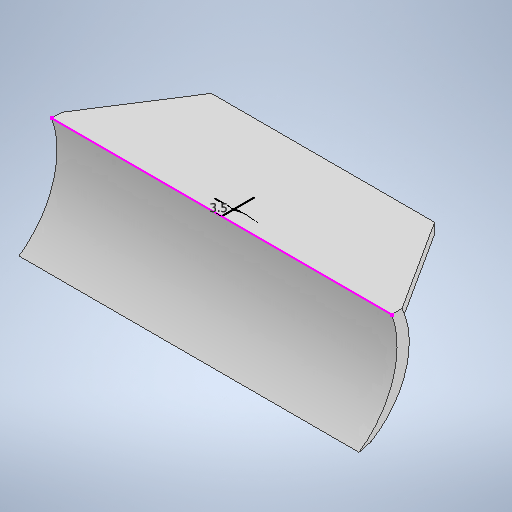
# Autodesk Inventor part: slope
Saved by Autodesk Inventor 2025.1 (Build 291241020, 241B)
## iProperties
Created: 2025-04-15
Part Number: slope
Material: Generic
Document SubType Name: Modeling
Designer: omiye
Density: 1 g/cm^3
Appearance: Default
Author: omiye
Autodesk Inventor part; units mm, degrees
ref_plane "YZ Plane" through (0, 0, 0) normal (1, 0, 0) x (0, 1, 0)
ref_plane "XZ Plane" through (0, 0, 0) normal (0, 1, 0) x (-1, 0, 0)
ref_plane "XY Plane" through (0, 0, 0) normal (0, 0, 1) x (1, 0, 0)
sketch "Sketch1" plane through (0, 0, 0) normal (0, 1, 0) x (-1, 0, 0)
  line L0 (0, 0) -> (32.5, 0)
  line L1 (32.5, 0) -> (-32.5, 0)
  line L2 (-32.5, 0) -> (-32.5, 19)
  line L3 (-32.5, 19) -> (32.5, 19)
  line L4 (32.5, 19) -> (32.5, 0)
  dimension "d0" = 32.5
  dimension "d1" = 65
  dimension "d2" = 19
  constraints: 10 end point, 2 perpendicular, 1 horizontal, 1 point on line, 1 vertical
  measures "d0" distance of L0.start L0.end
  measures "d1" distance of L0.end L1.end
  measures "d2" distance of L1.end L2.end
extrude "Extrusion1" add sketch "Sketch1" along normal blind 25
sketch "Sketch2" plane through (32.5, 0, 19) normal (1, 0, 0) x (0, 0, -1)
  line L0 (19, 0) -> (8, 0)
  line L1 (0, 0) -> (19, 0)
  line L2 (8, 0) -> (0, -2.143594)
  line L3 (0, -2.143594) -> (0, 0)
  dimension "d5" = 11
  dimension "d6" = 165
  constraints: 6 end point, 1 perpendicular, 1 point on line
  measures "d5" distance of L0.start L0.end
  measures "d6" angle of L2 L0
extrude "Extrusion2" add sketch "Sketch2" against normal up to surface (65 mm away)
sketch "Sketch3" plane through (32.5, 0, 0) normal (1, 0, 0) x (0, 0, -1)
  line L0 (-19, -2.143594) -> (-19, 25)
  line L1 (-19, 25) -> (0, 25)
  line L2 (-19, 25) -> (-19, -5)
  arc A0 (-19, -5) -> (-9.5, 25) centre (-33.73129, 16.169075) ccw
  line L3 (-19, -2.143594) -> (-11, 0)
  line L4 (-19, -5) -> (-11, 0)
  line L5 (-19, -2.143594) -> (-19, 25)
  line L6 (-19, 25) -> (-9.5, 25)
  point P0 (0, 0)
  point P1 (-14.409764, -0.913643)
  dimension "d59" = 30
  constraints: 8 end point, 2 midpoint, 2 point on circle, 1 centre point, 1 collinear, 1 perpendicular, 1 point on line
  measures "d59" distance of L0.end L2.end
extrude "Extrusion3" cut sketch "Sketch3" against normal blind 81.4375 contours L0 L1 A0 L3
sketch "Sketch4" plane through (0, 0, 0) normal (0, -1, 0) x (1, 0, 0)
  line L0 (-32.5, 0) -> (-32.5, 11) projected
  line L1 (-32.5, 0) -> (-32.5, 10.5)
  line L2 (-32.5, 10.5) -> (32.5, 10.5)
  line L3 (32.5, 11) -> (32.5, 0) projected
  line L4 (-32.5, 0) -> (-32.5, 5.25)
  line L5 (-32.5, 5.25) -> (32.5, 5.25)
  line L6 (-32.5, 5.25) -> (-18.75, 5.25)
  line L7 (-18.75, 5.25) -> (0, 5.25)
  line L8 (0, 5.25) -> (18.75, 5.25)
  line L9 (18.75, 5.25) -> (32.5, 5.25)
  circle A0 centre (18.75, 5.25) radius 1.525
  circle A1 centre (0, 5.25) radius 1.525
  circle A2 centre (-18.75, 5.25) radius 1.525
  point P0 (0, 0)
  point P1 (-17.225, 5.25)
  point P2 (-20.275, 5.25)
  point P3 (1.525, 5.25)
  point P4 (-1.525, 5.25)
  point P5 (20.275, 5.25)
  point P6 (17.225, 5.25)
  dimension "d12" = 10.5
  dimension "d13" = 5.25
  dimension "d14" = 13.75
  dimension "d15" = 18.75
  dimension "d16" = 18.75
  dimension "d17" = 3.05
  dimension "d18" = 3.05
  dimension "d19" = 3.05
  constraints: 16 end point, 5 point on line, 3 centre point, 3 coincident, 3 perpendicular, 2 midpoint
  measures "d12" distance of L0.start L1.end
  measures "d13" distance of L0.start L4.end
  measures "d14" distance of L4.end L6.end
  measures "d15" distance of L6.end L7.end
  measures "d16" distance of L7.end L8.end
  measures "d17" diameter of A0
  measures "d18" diameter of A1
  measures "d19" diameter of A2
extrude "Extrusion4" cut sketch "Sketch4" against normal blind 4 contours A2 L5 | L5 A2 | A1 L5 | L5 A1 | A0 L5 | L5 A0
sketch "Sketch5" plane through (32.5, 0, 0) normal (0, 0, -1) x (-1, 0, 0)
  line L0 (0, 25) -> (65, 25)
  line L1 (65, 25) -> (65, -2.143594)
  line L2 (0, 25) -> (65, 25)
  line L3 (65, 25) -> (65, 22)
  line L4 (65, 22) -> (0, 22)
  line L5 (0, 22) -> (0, 25)
  point P0 (32.5, 0)
  dimension "d22" = 3
  constraints: 8 end point, 2 parallel, 1 horizontal, 1 perpendicular, 1 point on line
  measures "d22" distance of L2.end L3.end
sketch "Sketch6" plane through (32.5, 0, 0) normal (1, 0, 0) x (0, 0, -1)
  line L0 (0, 0) -> (-11, 0)
  line L1 (0, 0) -> (-10, 0)
  line L2 (-11, 0) -> (0, 0)
  line L3 (-19, 25) -> (0, 25)
  arc A0 (-11, 0) -> (-6.906688, 25) centre (-24.791662, 15.093247) ccw
  line L4 (0, 0) -> (0, 25)
  line L5 (0, 25) -> (0, 22)
  line L6 (0, 22) -> (-5.548149, 22)
  line L7 (0, 0) -> (0, 2.5)
  line L8 (0, 2.5) -> (-8.68495, 2.5)
  point P0 (-9.5, 25)
  dimension "d23" = 10
  dimension "d24" = 3
  dimension "d25" = 2.5
  constraints: 10 end point, 4 point on circle, 4 point on line, 1 centre point, 1 horizontal, 1 perpendicular
  measures "d23" distance of L0.start L1.end
  measures "d24" distance of L3.end L5.end
  measures "d25" distance of L0.start L7.end
extrude "Extrusion5" cut sketch "Sketch6" against normal blind 113.5375 contours L8 A0 L6 L4
extrude "Extrusion6" add sketch "Sketch5" along normal blind 20
sketch "Sketch12" plane through (0, 25, 0) normal (0, 1, 0) x (1, 0, 0)
  line L0 (0, 0) -> (0, -9.5)
  line L1 (49.5, -9.5) -> (-49.5, -9.5)
  line L2 (0, -9.5) -> (0, 0)
  line L3 (0, -9.5) -> (0, -6)
  line L4 (0, -6) -> (8.228384, -6)
  line L5 (8.228384, -6) -> (-5.400421, -6)
  dimension "d85" = 3.5
  constraints: 10 end point, 2 point on line, 1 collinear, 1 midpoint, 1 perpendicular
  measures "d85" distance of L0.end L3.end
sketch "Sketch14" plane through (32.5, 0, 11) normal (1, 0, 0) x (0, 0, -1)
  line L0 (11, 0) -> (0, 0)
  line L1 (0, 0) -> (9.434, 0) construction
  arc A0 (-3.409764, -0.913643) -> (1.5, 25) centre (-22.73129, 16.169075) ccw
  line L2 (1.5, 25) -> (31, 25)
  arc A1 (-8.000486, -4.999258) -> (1.5, 25) centre (-22.726506, 16.168322) ccw
  line L3 (-3.409764, -0.913643) -> (0, 0)
  line L4 (-3.409764, -0.913643) -> (0, 0)
  line L5 (-8.000486, -4.999258) -> (-4.590768, -4.085627)
  line L6 (-8.000486, -4.999258) -> (-4.470486, -4.999258) construction
  line L7 (-4.590768, -4.085627) -> (0, 0)
  point P0 (28, 25)
  point P1 (-2.386043, 0.31942)
  dimension "d60" = 9.434
  dimension "d62" = 3.53
  dimension "d63" = 15
  constraints: 10 end point, 2 horizontal, 2 point on circle, 1 centre point, 1 collinear, 1 equal length
  measures "d60" distance of L0.end L5.start
  measures "d62" distance of L5.start L5.end
  measures "d63" angle of L6 L5
extrude "Extrusion12" add sketch "Sketch14" against normal up to surface (65 mm away)
sketch "Sketch15" plane through (32.5, 0, 0) normal (1, 0, 0) x (0, 0, -1)
  arc A0 (-19.000486, -4.999258) -> (-13.386043, 0.31942) centre (-33.726506, 16.168322) ccw
  line L0 (-9.5, 25) -> (20, 25)
  arc A1 (-19.000486, -4.999258) -> (-9.5, 25) centre (-33.729569, 16.169292) ccw
  line L1 (-9.5, 25) -> (-6.5, 25)
  line L2 (-19.000486, -4.999258) -> (-15.590768, -4.085627)
  arc A2 (-15.590768, -4.085627) -> (-6.5, 25) centre (-27.017687, 15.44936) ccw
  line L3 (-15.590768, -4.085627) -> (-11, 0)
  line L4 (-19.000486, -4.999258) -> (-15.590768, -4.085627)
  line L5 (-9.5, 25) -> (-6.5, 25)
  line L6 (-9.5, 25) -> (20, 25)
  point P0 (0, 0)
  point P1 (17, 25)
  dimension "d66" = 3
  constraints: 6 end point, 4 point on circle, 2 centre point, 2 collinear, 1 point on line
  measures "d66" distance of L0.start L1.end
extrude "Extrusion13" add sketch "Sketch15" against normal blind 65
sketch "Sketch16" plane through (32.5, 0, 0) normal (1, 0, 0) x (0, 0, -1)
  line L0 (-19.000486, -4.999258) -> (-15.590768, -4.085627)
  arc A0 (-8.067422, 13.618284) -> (-9.5, 25) centre (-33.73129, 16.169075) ccw
  arc A1 (-19.000486, -4.999258) -> (-9.5, 25) centre (-33.729569, 16.169292) ccw
  line L1 (-9.5, 25) -> (20, 25)
  line L2 (-9.5, 25) -> (-6.5, 25)
  arc A2 (-15.590768, -4.085627) -> (-10.479625, 0) centre (-27.017687, 15.44936) ccw
  arc A3 (-6.108674, 6.78891) -> (-4.450402, 17.154601) centre (-24.791662, 15.093247) ccw
  arc A4 (-15.590768, -4.085627) -> (-6.5, 25) centre (-27.017687, 15.44936) ccw
  line L3 (-19.000486, -4.999258) -> (-15.590768, -4.085627)
  line L4 (-9.5, 25) -> (-6.5, 25)
  point P0 (0, 0)
  point P1 (17, 25)
  point P2 (-10.479625, 0)
  dimension "d69" = 3
  constraints: 6 end point, 6 point on circle, 2 centre point, 2 collinear, 1 point on line
  measures "d69" distance of L1.start L2.end
sketch "Sketch16 outline for Extrusion14" plane through (32.5, 0, 0) normal (1, 0, 0) x (0, 0, -1)
  arc A0 (-10.479625, 0) -> (-6.5, 25) centre (-27.017687, 15.44936) ccw
  arc A1 (-15.590768, -4.085627) -> (-10.479625, 0) centre (-27.017687, 15.44936) ccw
  line L0 (-19.000486, -4.999258) -> (-15.590768, -4.085627)
  arc A2 (-9.5, 25) -> (-19.000486, -4.999258) centre (-33.729569, 16.169292) cw
  line L1 (-6.5, 25) -> (-9.5, 25)
extrude "Extrusion14" add sketch "Sketch16 outline for Extrusion14" along normal blind 17
sketch "Sketch17" plane through (-32.5, 0, 0) normal (-1, 0, 0) x (0, 0, 1)
  line L0 (9.5, 25) -> (-20, 25)
  line L1 (19.000486, -4.999258) -> (15.590768, -4.085627)
  arc A0 (8.067422, 13.618284) -> (19.000486, -4.999258) centre (33.729569, 16.169292) ccw
  arc A1 (9.5, 25) -> (19.000486, -4.999258) centre (33.729569, 16.169292) ccw
  line L2 (9.5, 25) -> (6.5, 25)
  arc A2 (4.450402, 17.154601) -> (6.108674, 6.78891) centre (24.791662, 15.093247) ccw
  arc A3 (6.5, 25) -> (15.590768, -4.085627) centre (27.017687, 15.44936) ccw
  line L3 (15.590768, -4.085627) -> (19.000486, -4.999258)
  point P0 (0, 0)
  point P1 (-17, 25)
  dimension "d72" = 3
  constraints: 6 point on circle, 4 end point, 2 centre point, 1 collinear, 1 point on line
  measures "d72" distance of L0.start L2.end
sketch "Sketch17 outline for Extrusion15" plane through (-32.5, 0, 0) normal (-1, 0, 0) x (0, 0, 1)
  arc A0 (6.5, 25) -> (15.590768, -4.085627) centre (27.017687, 15.44936) ccw
  line L0 (9.5, 25) -> (6.5, 25)
  arc A1 (8.067422, 13.618284) -> (9.5, 25) centre (33.729569, 16.169292) cw
  arc A2 (19.000486, -4.999258) -> (8.067422, 13.618284) centre (33.729569, 16.169292) cw
  line L1 (15.590768, -4.085627) -> (19.000486, -4.999258)
extrude "Extrusion15" add sketch "Sketch17 outline for Extrusion15" along normal blind 17
sketch "Sketch18" plane through (-32.5, 15.093247, 24.791662) normal (-1, 0, 0) x (0, 0.1579684, 0.9874442)
  arc A0 (-16.497042, 12.67187) -> (-18.101737, 9.890438) centre (2.25433, 0) ccw
  arc A1 (-18.11904, -9.854746) -> (-16.516593, -12.64289) centre (2.25433, 0) ccw
  arc A2 (-18.101737, 9.890438) -> (-18.11904, -9.854746) centre (2.25433, 0) ccw
  arc A3 (-19.76023, 5.248748) -> (-19.76023, -5.248748) centre (2.25433, 0) ccw
  arc A4 (-19.76023, 5.248748) -> (-19.76023, -5.248748) centre (0, 0) ccw
  point P0 (-26.864638, -10.98744)
  constraints: 4 point on circle, 2 centre point
sketch "Sketch18 outline for Extrusion16" plane through (-32.5, 15.093247, 24.791662) normal (-1, 0, 0) x (0, 0.1579684, 0.9874442)
  arc A0 (-19.76023, 5.248748) -> (-19.76023, -5.248748) centre (0, 0) ccw
  arc A1 (-19.76023, -5.248748) -> (-19.76023, 5.248748) centre (2.25433, 0) cw
extrude "Extrusion16" cut sketch "Sketch18 outline for Extrusion16" against normal blind 66.2125
sketch "Sketch20" plane through (0, 25, 0) normal (0, 1, 0) x (1, 0, 0)
  arc A0 (32.5, 17) -> (29.5, 20) centre (29.5, 17) ccw
  line L0 (32.5, -6.5) -> (49.5, -6.5)
  line L1 (-32.5, 20) -> (-32.5, -5.354831)
  line L2 (49.5, -6.5) -> (32.5, -6.5)
  line L3 (-32.5, -6.5) -> (-32.5, -5.354831)
  line L4 (-32.5, 17) -> (-32.5, -6.5)
  line L5 (-32.5, -6.5) -> (-49.5, -6.5)
  line L6 (32.5, -6.5) -> (32.5, 20)
  line L7 (32.5, 17) -> (32.5, -6.5)
  line L8 (32.5, 20) -> (49.5, -6.5)
  line L9 (-32.5, 20) -> (32.5, 20)
  line L10 (-32.5, 20) -> (-49.5, -6.5)
  point P0 (0, 0)
  constraints: 12 end point, 1 collinear, 1 horizontal, 1 perpendicular, 1 vertical
sketch "Sketch21" plane through (-49.5, 0, 0) normal (-1, 0, 0) x (0, 0, 1)
  arc A0 (9.5, 25) -> (19.000486, -4.999258) centre (33.729569, 16.169292) ccw
  line L0 (9.5, 25) -> (19.000486, -4.999258)
  point P0 (0, 0)
  constraints: 2 end point, 2 point on circle, 1 centre point
extrude "Extrusion18" cut sketch "Sketch21" against normal blind 124.3
extrude "Extrusion19" add sketch "Sketch20" against normal up to surface (3 mm away) contours L6 L8 L0 | L1 L3 L5 L10
body "Solid1"
